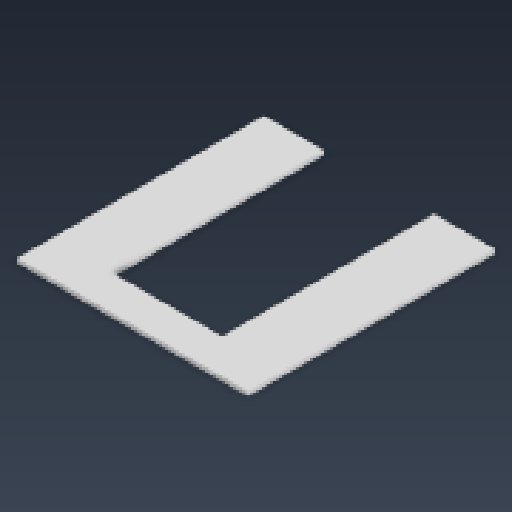
# Autodesk Inventor part: стульчак
Saved by Autodesk Inventor 2025 (Build 290162000, 162)
## iProperties
Created: 2025-01-28
Part Number: стульчак
Material: Типовые
Document SubType Name: Modeling
Designer: GameHD
Density: 1 g/cm^3
Appearance: По умолчанию
Author: GameHD
Autodesk Inventor part; units mm, degrees
ref_plane "YZ Plane" through (0, 0, 0) normal (1, 0, 0) x (0, 1, 0)
ref_plane "XZ Plane" through (0, 0, 0) normal (0, 1, 0) x (-1, 0, 0)
ref_plane "XY Plane" through (0, 0, 0) normal (0, 0, 1) x (1, 0, 0)
sketch "Эскиз1" plane through (0, 0, 0) normal (0, 1, 0) x (-1, 0, 0)
  line L0 (-115, 123) -> (115, 123)
  line L1 (115, 123) -> (115, -123)
  line L2 (115, -123) -> (-115, -123)
  line L3 (-115, -123) -> (-115, 123)
  line L4 (-115, 123) -> (115, -123) construction
  line L5 (115, 123) -> (-115, -123) construction
  point P0 (0, 0)
  dimension "d0" = 230
  dimension "d1" = 246
  constraints: 12 end point, 2 midpoint, 2 parallel, 1 horizontal, 1 perpendicular
  measures "d0" distance of L1.end L2.end
  measures "d1" distance of L0.end L1.end
extrude "Выдавливание1" add sketch "Эскиз1" along normal blind 4
sketch "Эскиз2" plane through (0, 0, 0) normal (0, -1, 0) x (1, 0, 0)
  line L0 (-65.9289, -30.8784) -> (-65.9289, 53.4389) projected
  line L1 (65.9289, -33.6328) -> (65.9289, 50.6846) projected
  line L2 (115, -123) -> (-115, -123) projected
  line L3 (-115, 123) -> (115, 123) projected
  line L4 (-115, -123) -> (-55, -123)
  line L5 (-55, -123) -> (-55, 123)
  line L6 (-55, 123) -> (-115, 123)
  line L7 (-115, 123) -> (-115, -123)
  line L8 (114.3, -123) -> (64.3, -123)
  line L9 (64.3, -123) -> (64.3, 123)
  line L10 (64.3, 123) -> (114.3, 123)
  line L11 (114.3, 123) -> (114.3, -123)
  line L12 (21.8052, 115.9865) -> (21.8052, 75.1678) projected
  line L13 (64.3, 123) -> (-55, 123)
  line L14 (-55, 123) -> (-55, 88)
  line L15 (-55, 88) -> (64.3, 88)
  line L16 (64.3, 88) -> (64.3, 123)
  line L17 (115, -123) -> (-115, -123) projected
  line L18 (115, 123) -> (115, -123) projected
  line L19 (-115, 123) -> (115, 123) projected
  line L20 (-115, -123) -> (-115, 123) projected
  point P0 (0, 0)
  point P1 (64.3, 88)
  point P2 (64.3, -123)
  dimension "d4" = 60
  dimension "d5" = 50
  dimension "d7" = 35
  constraints: 24 end point, 6 parallel, 3 horizontal, 3 perpendicular, 3 point on line, 1 vertical
  measures "d4" distance of L6.end L5.end
  measures "d5" distance of L9.end L10.end
  measures "d7" distance of L14.end L13.end
extrude "Выдавливание2" cut sketch "Эскиз2" against normal blind 4 contours L2 L5 L15 L9
sketch "Эскиз3" plane through (0, 0, 0) normal (0, -1, 0) x (1, 0, 0)
  point P0 (0, 0)
sketch "Эскиз4" plane through (0, 0, 0) normal (0, -1, 0) x (1, 0, 0)
  point P0 (0, 0)
sketch "Эскиз5" plane through (0, 0, 0) normal (0, -1, 0) x (1, 0, 0)
  line L0 (-55, 88) -> (-55, -123) projected
  line L1 (-55, 88) -> (-59, 88)
  line L2 (-59, 88) -> (-59, 78)
  line L3 (-59, 78) -> (-55, 78)
  line L4 (-55, 78) -> (-55, 88)
  line L5 (-55, 78) -> (-59, 78)
  line L6 (-59, 78) -> (-59, 68)
  line L7 (-59, 68) -> (-55, 68)
  line L8 (-55, 68) -> (-55, 78)
  line L9 (-55, 68) -> (-59, 68)
  line L10 (-59, 68) -> (-59, 58)
  line L11 (-59, 58) -> (-55, 58)
  line L12 (-55, 58) -> (-55, 68)
  line L13 (-55, 58) -> (-59, 58)
  line L14 (-59, 58) -> (-59, 48)
  line L15 (-59, 48) -> (-55, 48)
  line L16 (-55, 48) -> (-55, 58)
  line L17 (-55, 48) -> (-59, 48)
  line L18 (-59, 48) -> (-59, 38)
  line L19 (-59, 38) -> (-55, 38)
  line L20 (-55, 38) -> (-55, 48)
  line L21 (-55, 38) -> (-59, 38)
  line L22 (-59, 38) -> (-59, 28)
  line L23 (-59, 28) -> (-55, 28)
  line L24 (-55, 28) -> (-55, 38)
  line L25 (-55, 28) -> (-59, 28)
  line L26 (-59, 28) -> (-59, 18)
  line L27 (-59, 18) -> (-55, 18)
  line L28 (-55, 18) -> (-55, 28)
  line L29 (-55, 18) -> (-59, 18)
  line L30 (-59, 18) -> (-59, 8)
  line L31 (-59, 8) -> (-55, 8)
  line L32 (-55, 8) -> (-55, 18)
  line L33 (-55, 8) -> (-59, 8)
  line L34 (-59, 8) -> (-59, -2)
  line L35 (-59, -2) -> (-55, -2)
  line L36 (-55, -2) -> (-55, 8)
  line L37 (-55, -2) -> (-59, -2)
  line L38 (-59, -2) -> (-59, -12)
  line L39 (-59, -12) -> (-55, -12)
  line L40 (-55, -12) -> (-55, -2)
  line L41 (-55, -12) -> (-59, -12)
  line L42 (-59, -12) -> (-59, -22)
  line L43 (-59, -22) -> (-55, -22)
  line L44 (-55, -22) -> (-55, -12)
  line L45 (-55, -22) -> (-59, -22)
  line L46 (-59, -22) -> (-59, -32)
  line L47 (-59, -32) -> (-55, -32)
  line L48 (-55, -32) -> (-55, -22)
  line L49 (-55, -32) -> (-59, -32)
  line L50 (-59, -32) -> (-59, -42)
  line L51 (-59, -42) -> (-55, -42)
  line L52 (-55, -42) -> (-55, -32)
  line L53 (-55, -42) -> (-59, -42)
  line L54 (-59, -42) -> (-59, -52)
  line L55 (-59, -52) -> (-55, -52)
  line L56 (-55, -52) -> (-55, -42)
  line L57 (-55, -52) -> (-59, -52)
  line L58 (-59, -52) -> (-59, -62)
  line L59 (-59, -62) -> (-55, -62)
  line L60 (-55, -62) -> (-55, -52)
  line L61 (-55, -62) -> (-59, -62)
  line L62 (-59, -62) -> (-59, -72)
  line L63 (-59, -72) -> (-55, -72)
  line L64 (-55, -72) -> (-55, -62)
  line L65 (-55, -72) -> (-59, -72)
  line L66 (-59, -72) -> (-59, -82)
  line L67 (-59, -82) -> (-55, -82)
  line L68 (-55, -82) -> (-55, -72)
  line L69 (-55, -82) -> (-59, -82)
  line L70 (-59, -82) -> (-59, -92)
  line L71 (-59, -92) -> (-55, -92)
  line L72 (-55, -92) -> (-55, -82)
  line L73 (-55, -92) -> (-59, -92)
  line L74 (-59, -92) -> (-59, -102)
  line L75 (-59, -102) -> (-55, -102)
  line L76 (-55, -102) -> (-55, -92)
  line L77 (-55, -102) -> (-59, -102)
  line L78 (-59, -102) -> (-59, -112)
  line L79 (-55, -112) -> (-55, -102)
  line L80 (4.65, 88) -> (4.65, -60.325)
  line L81 (64.3, 88) -> (64.3, -123)
  line L82 (64.3, 88) -> (68.3, 88)
  line L83 (68.3, 88) -> (68.3, 78)
  line L84 (68.3, 78) -> (64.3, 78)
  line L85 (64.3, 78) -> (64.3, 88)
  line L86 (68.3, 68) -> (64.3, 68)
  line L87 (68.3, 78) -> (68.3, 68)
  line L88 (64.3, 78) -> (68.3, 78)
  line L89 (64.3, 68) -> (64.3, 78)
  line L90 (68.3, 58) -> (64.3, 58)
  line L91 (68.3, 68) -> (68.3, 58)
  line L92 (64.3, 68) -> (68.3, 68)
  line L93 (64.3, 58) -> (64.3, 68)
  line L94 (68.3, 48) -> (64.3, 48)
  line L95 (68.3, 58) -> (68.3, 48)
  line L96 (64.3, 58) -> (68.3, 58)
  line L97 (64.3, 48) -> (64.3, 58)
  line L98 (68.3, 38) -> (64.3, 38)
  line L99 (68.3, 48) -> (68.3, 38)
  line L100 (64.3, 48) -> (68.3, 48)
  line L101 (64.3, 38) -> (64.3, 48)
  line L102 (68.3, 28) -> (64.3, 28)
  line L103 (68.3, 38) -> (68.3, 28)
  line L104 (64.3, 38) -> (68.3, 38)
  line L105 (64.3, 28) -> (64.3, 38)
  line L106 (68.3, 18) -> (64.3, 18)
  line L107 (68.3, 28) -> (68.3, 18)
  line L108 (64.3, 28) -> (68.3, 28)
  line L109 (64.3, 18) -> (64.3, 28)
  line L110 (68.3, 8) -> (64.3, 8)
  line L111 (68.3, 18) -> (68.3, 8)
  line L112 (64.3, 18) -> (68.3, 18)
  line L113 (64.3, 8) -> (64.3, 18)
  line L114 (68.3, -2) -> (64.3, -2)
  line L115 (68.3, 8) -> (68.3, -2)
  line L116 (64.3, 8) -> (68.3, 8)
  line L117 (64.3, -2) -> (64.3, 8)
  line L118 (68.3, -12) -> (64.3, -12)
  line L119 (68.3, -2) -> (68.3, -12)
  line L120 (64.3, -2) -> (68.3, -2)
  line L121 (64.3, -12) -> (64.3, -2)
  line L122 (68.3, -22) -> (64.3, -22)
  line L123 (68.3, -12) -> (68.3, -22)
  line L124 (64.3, -12) -> (68.3, -12)
  line L125 (64.3, -22) -> (64.3, -12)
  line L126 (68.3, -32) -> (64.3, -32)
  line L127 (68.3, -22) -> (68.3, -32)
  line L128 (64.3, -22) -> (68.3, -22)
  line L129 (64.3, -32) -> (64.3, -22)
  line L130 (68.3, -42) -> (64.3, -42)
  line L131 (68.3, -32) -> (68.3, -42)
  line L132 (64.3, -32) -> (68.3, -32)
  line L133 (64.3, -42) -> (64.3, -32)
  line L134 (68.3, -52) -> (64.3, -52)
  line L135 (68.3, -42) -> (68.3, -52)
  line L136 (64.3, -42) -> (68.3, -42)
  line L137 (64.3, -52) -> (64.3, -42)
  line L138 (68.3, -62) -> (64.3, -62)
  line L139 (68.3, -52) -> (68.3, -62)
  line L140 (64.3, -52) -> (68.3, -52)
  line L141 (64.3, -62) -> (64.3, -52)
  line L142 (68.3, -72) -> (64.3, -72)
  line L143 (68.3, -62) -> (68.3, -72)
  line L144 (64.3, -62) -> (68.3, -62)
  line L145 (64.3, -72) -> (64.3, -62)
  line L146 (68.3, -82) -> (64.3, -82)
  line L147 (68.3, -72) -> (68.3, -82)
  line L148 (64.3, -72) -> (68.3, -72)
  line L149 (64.3, -82) -> (64.3, -72)
  line L150 (68.3, -92) -> (64.3, -92)
  line L151 (68.3, -82) -> (68.3, -92)
  line L152 (64.3, -82) -> (68.3, -82)
  line L153 (64.3, -92) -> (64.3, -82)
  line L154 (68.3, -102) -> (64.3, -102)
  line L155 (68.3, -92) -> (68.3, -102)
  line L156 (64.3, -92) -> (68.3, -92)
  line L157 (64.3, -102) -> (64.3, -92)
  line L158 (68.3, -102) -> (68.3, -112)
  line L159 (64.3, -102) -> (68.3, -102)
  line L160 (64.3, -112) -> (64.3, -102)
  point P0 (0, 0)
  point P1 (64.3, 28)
  point P2 (64.3, -102)
  point P3 (64.3, -32)
  dimension "d10" = 4
  dimension "d11" = 10
  dimension "d12" = 4
  dimension "d13" = 10
  dimension "d14" = 4
  dimension "d15" = 10
  dimension "d16" = 4
  dimension "d17" = 10
  dimension "d18" = 4
  dimension "d19" = 10
  dimension "d20" = 4
  dimension "d21" = 10
  dimension "d22" = 4
  dimension "d23" = 10
  dimension "d24" = 4
  dimension "d25" = 10
  dimension "d26" = 4
  dimension "d27" = 10
  dimension "d28" = 4
  dimension "d29" = 10
  dimension "d30" = 4
  dimension "d31" = 10
  dimension "d32" = 4
  dimension "d33" = 10
  dimension "d34" = 4
  dimension "d35" = 10
  dimension "d36" = 4
  dimension "d37" = 10
  dimension "d38" = 4
  dimension "d39" = 10
  dimension "d40" = 4
  dimension "d41" = 10
  dimension "d42" = 4
  dimension "d43" = 10
  dimension "d44" = 4
  dimension "d45" = 10
  dimension "d46" = 4
  dimension "d47" = 10
  dimension "d49" = 10
  constraints: 320 end point, 80 symmetric about line, 39 parallel, 20 horizontal, 20 perpendicular, 1 vertical, 1 other
  measures "d10" distance of L3.end L2.end
  measures "d11" distance of L2.end L1.end
  measures "d12" distance of L7.end L7.start
  measures "d13" distance of L7.start L6.start
  measures "d14" distance of L11.end L11.start
  measures "d15" distance of L11.start L10.start
  measures "d16" distance of L15.end L15.start
  measures "d17" distance of L15.start L14.start
  measures "d18" distance of L19.end L19.start
  measures "d19" distance of L19.start L18.start
  measures "d20" distance of L23.end L23.start
  measures "d21" distance of L23.start L22.start
  measures "d22" distance of L27.end L27.start
  measures "d23" distance of L27.start L26.start
  measures "d24" distance of L31.end L31.start
  measures "d25" distance of L31.start L30.start
  measures "d26" distance of L35.end L35.start
  measures "d27" distance of L35.start L34.start
  measures "d28" distance of L39.end L39.start
  measures "d29" distance of L39.start L38.start
  measures "d30" distance of L43.end L43.start
  measures "d31" distance of L43.start L42.start
  measures "d32" distance of L47.end L47.start
  measures "d33" distance of L47.start L46.start
  measures "d34" distance of L51.end L51.start
  measures "d35" distance of L51.start L50.start
  measures "d36" distance of L55.end L55.start
  measures "d37" distance of L55.start L54.start
  measures "d38" distance of L59.end L59.start
  measures "d39" distance of L59.start L58.start
  measures "d40" distance of L63.end L63.start
  measures "d41" distance of L63.start L62.start
  measures "d42" distance of L67.end L67.start
  measures "d43" distance of L67.start L66.start
  measures "d44" distance of L71.end L71.start
  measures "d45" distance of L71.start L70.start
  measures "d46" distance of L75.end L75.start
  measures "d47" distance of L75.start L74.start
  measures "d49" distance of L78.end L78.start
extrude "Выдавливание3" cut sketch "Эскиз5" against normal blind 4 contours L0 L3 L2 L1 | L0 L11 L10 L7 | L0 L19 L18 L15 | L0 L27 L26 L23 | L0 L35 L34 L31 | L0 L43 L42 L39 | L0 L51 L50 L47 | L0 L59 L58 L55 | L0 L67 L66 L63 | L0 L75 L74 L71 | L82 L83 L84 L81 | L86 L91 L90 L81 | L94 L99 L98 L81 | L102 L107 L106 L81 | L110 L115 L114 L81 | L118 L123 L122 L81 | L126 L131 L130 L81 | L134 L139 L138 L81 | L142 L147 L146 L81 | L150 L155 L154 L81
sketch "Эскиз6" plane through (0, 0, 0) normal (0, -1, 0) x (1, 0, 0)
  line L0 (-115, -123) -> (-115, 123) projected
  line L1 (-115, 123) -> (-105, 123)
  line L2 (-115, 123) -> (115, 123) projected
  line L3 (-105, 123) -> (-105, -139.0315)
  circle A0 centre (-105, 79.375) radius 2.1
  circle A1 centre (-104.775, 0) radius 2.1
  circle A2 centre (-105, -96.8375) radius 2.1
  line L4 (0, 123) -> (0, -68.2625)
  circle A3 centre (105, 79.375) radius 2.1
  circle A4 centre (104.775, 0) radius 2.1
  circle A5 centre (105, -96.8375) radius 2.1
  line L5 (105, 123) -> (105, -139.0315)
  point P0 (0, 0)
  dimension "d79" = 10
  dimension "d80" = 4.2
  dimension "d81" = 4.2
  dimension "d82" = 4.2
  constraints: 8 end point, 6 centre point, 5 symmetric about line, 3 point on line, 1 midpoint, 1 perpendicular, 1 vertical, 3 other
  measures "d79" distance of L0.end L1.end
  measures "d80" diameter of A0
  measures "d81" diameter of A1
  measures "d82" diameter of A2
extrude "Выдавливание4" cut sketch "Эскиз6" against normal blind 4.2
equation "\"d52\" = d16"
